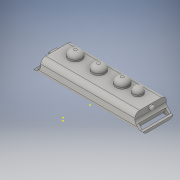
# Autodesk Inventor part: Hackathon
Saved by Autodesk Inventor 2016 (Build 200138000, 138)
## iProperties
Created: 2016-01-17
Part Number: Hackathon
Material: Generic
Document SubType Name: Modeling
Designer: Aditya
Density: 1 g/cm^3
Appearance: Default
Author: Aditya
Autodesk Inventor part; units mm, degrees
ref_plane "YZ Plane" through (0, 0, 0) normal (1, 0, 0) x (0, 1, 0)
ref_plane "XZ Plane" through (0, 0, 0) normal (0, 1, 0) x (-1, 0, 0)
ref_plane "XY Plane" through (0, 0, 0) normal (0, 0, 1) x (1, 0, 0)
sketch "Sketch1" plane through (0, 0, 0) normal (0, 1, 0) x (-1, 0, 0)
  line L0 (39.7631, -21.9226) -> (-36.4369, -21.9226)
  line L1 (-36.4369, -21.9226) -> (-36.4369, -47.3226)
  line L2 (-36.4369, -47.3226) -> (39.7631, -47.3226)
  line L3 (39.7631, -47.3226) -> (39.7631, -21.9226)
  point P0 (0, 0)
  dimension "d0" = 76.2
  dimension "d1" = 25.4
  constraints: 8 end point, 2 parallel, 1 horizontal, 1 perpendicular
  measures "d0" distance of L1.end L2.end
  measures "d1" distance of L2.end L0.start
extrude "Extrusion1" add sketch "Sketch1" along normal blind 12.7
sketch "Sketch2" plane through (0, 0, 0) normal (0, -1, 0) x (1, 0, 0)
  point P0 (0, 0)
sketch "Sketch3" plane through (0, 0, 0) normal (0, -1, 0) x (1, 0, 0)
  point P0 (0, 0)
sketch "Sketch4" plane through (36.4369, 0, -21.9226) normal (1, 0, 0) x (0, 0, -1)
  line L0 (0, 0) -> (25.4, 0)
  line L1 (25.4, 0) -> (25.4, 2.032)
  line L2 (25.4, 2.032) -> (0, 2.032)
  line L3 (0, 2.032) -> (0, 0)
  line L4 (25.4, 0) -> (25.4, 12.7) projected
  line L5 (0, 0) -> (25.4, 0) projected
  point P0 (-21.9226, 0)
  dimension "d4" = 25.4
  dimension "d5" = 0
  dimension "d6" = 0
  dimension "d7" = 2.032
  constraints: 8 end point, 2 parallel, 1 horizontal, 1 perpendicular
  measures "d4" distance of L1.end L2.end
  measures "d5" distance between parallel lines of L4 L1
  measures "d6" distance between parallel lines of L5 L0
  measures "d7" distance of L2.end L0.start
extrude "Extrusion2" add sketch "Sketch4" along normal blind 6.096
sketch "Sketch5" plane through (36.4369, 2.032, -21.9226) normal (0, 1, 0) x (1, 0, 0)
  line L0 (1.1363, 23.495) -> (4.191, 23.495)
  line L1 (4.191, 23.495) -> (4.191, 1.905)
  line L2 (4.191, 1.905) -> (1.1363, 1.905)
  line L3 (1.1363, 1.905) -> (1.1363, 23.495)
  line L4 (6.096, 25.4) -> (6.096, 0) projected
  line L5 (0, 0) -> (6.096, 0) projected
  point P0 (-36.4369, -21.9226)
  dimension "d10" = 21.59
  dimension "d11" = 1.905
  dimension "d12" = 1.905
  dimension "d13" = 3.0547
  constraints: 8 end point, 2 parallel, 1 horizontal, 1 perpendicular
  measures "d10" distance of L0.end L1.end
  measures "d11" distance between parallel lines of L4 L1
  measures "d12" distance between parallel lines of L5 L2
  measures "d13" distance of L0.start L0.end
extrude "Extrusion3" cut sketch "Sketch5" against normal blind 6.096
chamfer "Chamfer1" distance 4.064 angle 45 1 edges at (36.4369, 2.032, -34.6226)
fillet "Fillet1" radius 4.318 1 edges at (36.4369, 6.096, -34.6226)
chamfer "Chamfer2" distance 2.54 angle 45 1 edges at (37.5732, 0, -34.6226)
sketch "Sketch6" plane through (-39.7631, 0, -47.3226) normal (-1, 0, 0) x (0, 0, 1)
  line L0 (0, 0) -> (25.4, 0) projected
  line L1 (-0.0106, 2.032) -> (25.4, 2.032)
  line L2 (25.4, 2.032) -> (25.4, 0)
  line L3 (25.4, 0) -> (-0.0106, 0)
  line L4 (-0.0106, 0) -> (-0.0106, 2.032)
  point P0 (47.3226, 0)
  dimension "d23" = 2.032
  constraints: 8 end point, 2 parallel, 1 horizontal, 1 perpendicular
  measures "d23" distance of L1.end L0.end
extrude "Extrusion4" add sketch "Sketch6" along normal blind 6.096
sketch "Sketch7" plane through (-39.7631, 2.032, -21.9226) normal (0, 1, 0) x (1, 0, 0)
  line L0 (-1.016, 23.495) -> (-4.064, 23.495)
  line L1 (-4.064, 23.495) -> (-4.064, 1.905)
  line L2 (-4.064, 1.905) -> (-1.016, 1.905)
  line L3 (-1.016, 1.905) -> (-1.016, 23.495)
  line L4 (-6.096, 25.4106) -> (-6.096, 0) projected
  line L5 (-6.096, 0) -> (82.296, 0) projected
  point P0 (39.7631, -21.9226)
  dimension "d26" = 21.59
  dimension "d27" = 2.032
  dimension "d28" = 3.048
  dimension "d29" = 1.905
  constraints: 8 end point, 2 parallel, 1 horizontal, 1 perpendicular
  measures "d26" distance of L2.end L0.start
  measures "d27" distance between parallel lines of L4 L1
  measures "d28" distance of L1.end L2.end
  measures "d29" distance between parallel lines of L5 L2
sketch "Sketch8" plane through (-39.7631, 2.032, -21.9226) normal (0, 1, 0) x (1, 0, 0)
  point P0 (39.7631, -21.9226)
extrude "Extrusion5" cut sketch "Sketch7" against normal blind 6.096
chamfer "Chamfer3" distance 3.81 angle 45 1 edges at (-39.7631, 2.032, -34.6226)
fillet "Fillet2" radius 4.318 1 edges at (-39.7631, 5.842, -34.6226)
chamfer "Chamfer4" distance 3.81 angle 45 1 edges at (-40.7791, 0, -34.6226)
sketch "Sketch9" plane through (0, 12.7, 0) normal (0, 1, 0) x (1, 0, 0)
  circle A0 centre (23.7369, 37.1626) radius 3.81
  line L0 (-39.7631, 21.9226) -> (36.4369, 21.9226) projected
  line L1 (36.4369, 21.9226) -> (36.4369, 47.3226) projected
  circle A1 centre (11.0369, 37.1626) radius 5.08
  circle A2 centre (-8.0131, 37.1626) radius 5.08
  circle A3 centre (-27.0631, 37.1626) radius 5.08
  point P0 (0, 0)
  dimension "d39" = 7.62
  dimension "d40" = 15.24
  dimension "d41" = 12.7
  dimension "d42" = 10.16
  dimension "d43" = 25.4
  dimension "d44" = 10.16
  dimension "d45" = 44.45
  dimension "d46" = 10.16
  dimension "d47" = 63.5
  constraints: 4 centre point
  measures "d39" diameter of A0
  measures "d40" distance from line of L0 A0.centre
  measures "d41" distance from line of L1 A0.centre
  measures "d42" diameter of A1
  measures "d43" distance from line of L1 A1.centre
  measures "d44" diameter of A2
  measures "d45" distance from line of L1 A2.centre
  measures "d46" diameter of A3
  measures "d47" distance from line of L1 A3.centre
extrude "Extrusion6" add sketch "Sketch9" along normal blind 5.08
fillet "Fillet3" radius 3.81 4 edges at (19.9269, 17.78, -37.1626) (5.9569, 17.78, -37.1626) (-13.0931, 17.78, -37.1626) (-32.1431, 17.78, -37.1626)
sketch "Sketch10" plane through (36.4369, 12.7, -47.3226) normal (0, 0, -1) x (-1, 0, 0)
  circle A0 centre (21.9344, -6.35) radius 1.8701
  line L0 (82.296, -12.7) -> (-6.096, -12.7) projected
  point P0 (36.4369, -12.7)
  dimension "d51" = 6.35
  constraints: 1 centre point
  measures "d51" distance from line of L0 A0.centre
extrude "Extrusion7" cut sketch "Sketch10" against normal blind 5.08
sketch "Sketch11" plane through (36.4369, 12.7, -47.3226) normal (0, 0, -1) x (-1, 0, 0)
  line L0 (26.8351, -6.1595) -> (28.0769, -5.207)
  line L1 (28.0769, -5.207) -> (33.3262, -5.207)
  line L2 (33.3262, -5.207) -> (34.4551, -6.1595)
  line L3 (34.4551, -6.1595) -> (34.4551, -7.112)
  line L4 (34.4551, -7.112) -> (26.8351, -7.112)
  line L5 (26.8351, -7.112) -> (26.8351, -6.1595)
  line L6 (82.296, -12.7) -> (-6.096, -12.7) projected
  point P0 (36.4369, -12.7)
  dimension "d54" = 0.9525
  dimension "d55" = 0.9525
  dimension "d56" = 0.9525
  dimension "d57" = 7.62
  dimension "d58" = 0.9525
  dimension "d59" = 5.588
  constraints: 12 end point, 2 perpendicular, 1 horizontal, 1 point on line, 1 vertical
  measures "d54" vertical distance of L1.end L2.end
  measures "d55" vertical distance of L0.start L0.end
  measures "d56" distance of L4.end L5.end
  measures "d57" distance of L3.end L4.end
  measures "d58" distance of L2.end L3.end
  measures "d59" distance between parallel lines of L6 L4
extrude "Extrusion8" cut sketch "Sketch11" against normal blind 3.81
sketch "Sketch12" plane through (-39.7631, 12.7, -47.3226) normal (-1, 0, 0) x (0, 0, 1)
  line L0 (10.0947, -1.27) -> (16.4447, -1.27)
  line L1 (16.4447, -1.27) -> (16.4447, -3.81)
  line L2 (16.4447, -3.81) -> (10.0947, -3.81)
  line L3 (10.0947, -3.81) -> (10.0947, -1.27)
  line L4 (0, 0) -> (25.4, 0) projected
  point P0 (47.3226, -12.7)
  dimension "d62" = 6.35
  dimension "d63" = 2.54
  dimension "d64" = 1.27
  constraints: 8 end point, 2 parallel, 1 horizontal, 1 perpendicular
  measures "d62" distance of L0.start L0.end
  measures "d63" distance of L0.end L1.end
  measures "d64" distance between parallel lines of L4 L0
extrude "Extrusion9" add sketch "Sketch12" along normal blind 2.54
fillet "Fillet4" radius 3.81 2 edges at (-1.6631, 12.7, -21.9226) (-1.6631, 12.7, -47.3226)
fillet "Fillet5" radius 3.81 2 edges at (1.3849, 0, -47.3226) (-1.6631, 0, -21.9226)
sketch "Sketch13" plane through (36.4369, 7.8846, -21.9226) normal (1, 0, 0) x (0, 0, -1)
  circle A0 centre (12.7, 2.7078) radius 1.7024
  line L0 (15.3053, 1.0054) -> (8.9553, 1.0054) projected
  arc A1 (3.81, 4.8154) -> (0, 1.0054) centre (3.81, 1.0054) ccw projected
  point P0 (-21.9226, -7.8846)
  dimension "d69" = 8.89
  constraints: 1 centre point, 1 tangent
  measures "d69" horizontal distance of A1.centre A0.centre
extrude "Extrusion10" add sketch "Sketch13" along normal blind 2.54
fillet "Fillet6" radius 1.651 1 edges at (38.9769, 10.5924, -32.9203)
sketch "Sketch14" plane through (-39.7631, 8.89, -21.9226) normal (0, 0, 1) x (1, 0, 0)
  point P0 (39.7631, -8.89)
sketch "Sketch15" plane through (40.6279, 2.032, -23.8276) normal (0, 1, 0) x (1, 0, 0)
  point P0 (-40.6279, -23.8276)
sketch "Sketch16" plane through (-43.8271, 2.032, -23.8276) normal (0, 1, 0) x (1, 0, 0)
  point P0 (43.8271, -23.8276)
body "Solid1"
